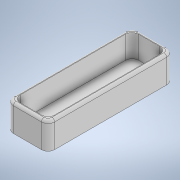
# Autodesk Inventor part: Support
Saved by Autodesk Inventor 2022 (Build 260153000, 153)
## iProperties
Created: 2022-05-11
Part Number: Support
Material: Générique
Document SubType Name: Modeling
Designer: timot
Density: 1 g/cm^3
Appearance: Par défaut
Author: timot
Autodesk Inventor part; units mm, degrees
ref_plane "YZ Plane" through (0, 0, 0) normal (1, 0, 0) x (0, 1, 0)
ref_plane "XZ Plane" through (0, 0, 0) normal (0, 1, 0) x (-1, 0, 0)
ref_plane "XY Plane" through (0, 0, 0) normal (0, 0, 1) x (1, 0, 0)
sketch "Esquisse1" plane through (0, 0, 0) normal (0, 1, 0) x (-1, 0, 0)
  line L0 (10.5, 47) -> (-10.5, 47)
  line L1 (-15.5, 42) -> (-15.5, -42)
  line L2 (-10.5, -47) -> (10.5, -47)
  line L3 (15.5, -42) -> (15.5, 42)
  line L4 (15.5, 47) -> (-15.5, -47) construction
  line L5 (-15.5, 47) -> (15.5, -47) construction
  arc A0 (15.5, 42) -> (10.5, 47) centre (10.5, 42) ccw
  arc A1 (-10.5, 47) -> (-15.5, 42) centre (-10.5, 42) ccw
  arc A2 (-15.5, -42) -> (-10.5, -47) centre (-10.5, -42) ccw
  arc A3 (10.5, -47) -> (15.5, -42) centre (10.5, -42) ccw
  point P0 (0, 0)
  dimension "d0" = 31
  dimension "d1" = 94
  dimension "d2" = 5
  constraints: 12 end point, 8 point on circle, 8 point on line, 8 tangent, 4 centre point, 3 equal radius, 2 midpoint, 2 parallel, 1 horizontal, 1 perpendicular
  measures "d0" distance of L5.end L4.end
  measures "d1" distance of L4.end L5.start
  measures "d2" radius of A0
sketch "Esquisse2" plane through (0, 0, 0) normal (0, 1, 0) x (-1, 0, 0)
  point P0 (0, 0)
extrude "Extrusion1" add sketch "Esquisse1" along normal blind 20
sketch "Esquisse3" plane through (0, 20, 0) normal (0, 1, 0) x (1, 0, 0)
  line L0 (-8, -44.5) -> (8, -44.5)
  line L1 (13, -39.5) -> (13, 39.5)
  line L2 (8, 44.5) -> (-8, 44.5)
  line L3 (-13, 39.5) -> (-13, -39.5)
  line L4 (-13, -44.5) -> (13, 44.5) construction
  line L5 (13, -44.5) -> (-13, 44.5) construction
  arc A0 (-13, -39.5) -> (-8, -44.5) centre (-8, -39.5) ccw
  arc A1 (-8, 44.5) -> (-13, 39.5) centre (-8, 39.5) ccw
  arc A2 (13, 39.5) -> (8, 44.5) centre (8, 39.5) ccw
  arc A3 (8, -44.5) -> (13, -39.5) centre (8, -39.5) ccw
  circle A4 centre (0, 30) radius 1.5
  line L6 (-13, 0) -> (13, 0)
  circle A5 centre (0, -30) radius 1.5
  point P0 (0, 0)
  dimension "d5" = 26
  dimension "d6" = 89
  dimension "d7" = 5
  dimension "d10" = 3
  dimension "d11" = 30
  constraints: 14 end point, 8 point on circle, 8 point on line, 8 tangent, 6 centre point, 4 midpoint, 3 equal radius, 2 parallel, 1 horizontal, 1 perpendicular, 1 symmetric about line, 1 other
  measures "d5" distance of L5.end L4.end
  measures "d6" distance of L4.end L5.start
  measures "d7" radius of A0
  measures "d10" diameter of A4
  measures "d11" distance of point (0, 0) A4.centre
extrude "Extrusion2" cut sketch "Esquisse3" against normal blind 17 contours A0 L3 L6 L1 A3 L0 | L3 A1 L2 A2 L1 L6 | A4 | A5
extrude "Extrusion3" cut sketch "Esquisse3" against normal blind 20 contours A4 | A5
chamfer "Chanfrein1" distance 2 angle 45 2 edges at (-1.5, 3, -30) (-1.5, 3, 30)
fillet "Congé1" radius 2 8 edges at (-15.5, 20, 0) (-14.0355, 20, 45.5355) (0, 20, 47) (14.0355, 20, 45.5355) (15.5, 20, 0) (14.0355, 20, -45.5355) (0, 20, -47) (-14.0355, 20, -45.5355)
